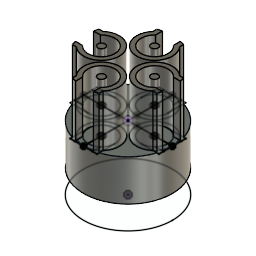
hexbug_circle_station (Autodesk Fusion 360 design; units mm, degrees)
Autodesk Fusion 360 part; units mm, degrees
note: some values were not read from the file. Set by a fixed rule: which sketch regions a step uses.
sketch "Sketch1" plane through (0, 0, 0) normal (0, 0, 1) x (1, 0, 0)
  circle A0 centre (0, 0) radius 12.45
  dimension "d1" = 24.9
  constraint coincident A0.centre origin
  measures "d1" diameter of A0
extrude "Extrude1" add sketch "Sketch1" along normal blind 18
sketch "Sketch2" plane through (0, 0, 18) normal (0, 0, 1) x (-1, 0, 0)
  circle A0 centre (0, 0) radius 12.45
  line L0 (0, 0) -> (0, -12.45)
  line L1 (0, 0) -> (-12.45, 0)
  line L2 (0, 0) -> (0, 12.45)
  line L3 (0, 0) -> (12.45, 0)
  line L4 (-12.45, 0) -> (-2.45, 0)
  circle A1 centre (-7.45, 0) radius 5
  line L5 (12.45, 0) -> (2.45, 0)
  line L6 (0, 12.45) -> (0, 2.45)
  line L7 (0, -12.45) -> (0, -2.45)
  circle A2 centre (0, -7.45) radius 5
  circle A3 centre (7.45, 0) radius 5
  circle A4 centre (0, 7.45) radius 5
  circle A5 centre (-7.45, 0) radius 3.75
  circle A6 centre (0, -7.45) radius 3.75
  circle A7 centre (0, 7.45) radius 3.75
  circle A8 centre (7.45, 0) radius 3.75
  circle A9 centre (-7.45, 0) radius 1
  circle A10 centre (0, -7.45) radius 1
  circle A11 centre (0, 7.45) radius 1
  circle A12 centre (7.45, 0) radius 1
  line L8 (-12.45, 0) -> (-12.45, -2.5)
  line L9 (-12.45, 0) -> (-12.45, 2.5)
  line L10 (-12.45, 2.5) -> (-11.7801, 2.5)
  line L11 (-12.45, -2.5) -> (-11.7801, -2.5)
  line L12 (0, -12.45) -> (-2.5, -12.45)
  line L13 (0, -12.45) -> (2.5, -12.45)
  line L14 (-2.5, -12.45) -> (-2.5, -11.7801)
  line L15 (12.45, 0) -> (12.45, -2.5)
  line L16 (12.45, 0) -> (12.45, 2.5)
  line L17 (12.45, 2.5) -> (10.2451, 2.5)
  line L18 (12.45, -2.5) -> (10.2451, -2.5)
  line L19 (2.5, -12.45) -> (2.5, -11.7801)
  line L20 (-2.5, -12.45) -> (-3.75, -12.45)
  line L21 (-3.75, -12.45) -> (-3.75, -10.7572)
  line L22 (2.5, -12.45) -> (3.75, -12.45)
  line L23 (3.75, -12.45) -> (3.75, -10.7572)
  line L24 (-3.75, -10.7572) -> (-3.75, -7.45)
  line L25 (2.5, -11.7801) -> (2.5, -10.2451)
  line L26 (-2.5, -11.7801) -> (-2.5, -10.2451)
  line L27 (3.75, -10.7572) -> (3.75, -7.45)
  line L28 (12.45, -2.5) -> (12.45, -3.75)
  line L29 (12.45, -3.75) -> (7.45, -3.75)
  line L30 (12.45, 1.25) -> (12.45, 2.5)
  line L31 (12.45, 2.5) -> (10.2451, 2.5)
  line L32 (12.45, 2.5) -> (12.45, 3.75)
  line L33 (12.45, 3.75) -> (7.45, 3.75)
  line L34 (0, 12.45) -> (-2.5, 12.45)
  line L35 (0, 12.45) -> (2.5, 12.45)
  line L36 (2.5, 12.45) -> (2.5, 10.2451)
  line L37 (2.5, 12.45) -> (3.75, 12.45)
  line L38 (3.75, 12.45) -> (3.75, 7.45)
  line L39 (-3.75, 7.45) -> (-3.75, 12.45)
  line L40 (-3.75, 12.45) -> (-2.5, 12.45)
  line L41 (-2.5, 12.45) -> (-2.5, 10.2451)
  line L42 (-11.7801, 2.5) -> (-10.2451, 2.5)
  line L43 (-11.7801, -2.5) -> (-10.2451, -2.5)
  line L44 (-12.45, -2.5) -> (-12.45, -3.75)
  line L45 (-12.45, 2.5) -> (-12.45, 3.75)
  line L46 (-12.45, 3.75) -> (-7.45, 3.75)
  line L47 (-12.45, -3.75) -> (-7.45, -3.75)
  dimension "d4" = 10
  dimension "d5" = 10
  dimension "d6" = 10
  dimension "d7" = 10
  dimension "d8" = 7.5
  dimension "d9" = 7.5
  dimension "d10" = 7.5
  dimension "d11" = 7.5
  dimension "d12" = 2
  dimension "d13" = 2
  dimension "d14" = 2
  dimension "d15" = 2
  dimension "d16" = 2.5
  dimension "d17" = 2.5
  dimension "d18" = 2.5
  dimension "d19" = 2.5
  dimension "d20" = 2.5
  dimension "d21" = 2.5
  dimension "d22" = 1.25
  dimension "d23" = 1.25
  dimension "d24" = 1.25
  dimension "d26" = 1.25
  dimension "d31" = 2.5
  dimension "d32" = 2.5
  dimension "d33" = 1.25
  dimension "d36" = 1.25
  dimension "d37" = 1.25
  constraint coincident A0.centre L0.start
  constraint coincident A0 L0.end
  constraint vertical L0
  constraint coincident A0 L1.end
  constraint perpendicular L0 L1
  constraint coincident A0 L2.end
  constraint perpendicular L1 L2
  constraint coincident A0 L3.end
  constraint perpendicular L2 L3
  constraint parallel L1 L4
  constraint midpoint L4 A1.centre
  constraint coincident L1.end A1
  constraint parallel L3 L5
  constraint parallel L2 L6
  constraint parallel L0 L7
  constraint midpoint L7 A2.centre
  constraint coincident L0.end A2
  constraint midpoint L5 A3.centre
  constraint coincident L3.end A3
  constraint midpoint L6 A4.centre
  constraint coincident L6.end A4
  constraint concentric A1 A5
  constraint concentric A2 A6
  constraint concentric A4 A7
  constraint concentric A3 A8
  constraint concentric A1 A9
  constraint concentric A6 A10
  constraint concentric A7 A11
  constraint concentric A8 A12
  constraint perpendicular L1 L8
  constraint perpendicular L1 L9
  constraint coincident A1 L10.end
  constraint perpendicular L9 L10
  constraint coincident A1 L11.end
  constraint perpendicular L8 L11
  constraint perpendicular L0 L12
  constraint perpendicular L0 L13
  constraint coincident A2 L14.end
  constraint perpendicular L12 L14
  constraint perpendicular L3 L15
  constraint perpendicular L3 L16
  constraint coincident A8 L17.end
  constraint perpendicular L16 L17
  constraint coincident A8 L18.end
  constraint perpendicular L15 L18
  constraint coincident A2 L19.end
  constraint perpendicular L13 L19
  constraint perpendicular L14 L20
  constraint coincident A2 L21.end
  constraint perpendicular L20 L21
  constraint perpendicular L19 L22
  constraint coincident A2 L23.end
  constraint perpendicular L22 L23
  constraint coincident A6 L24.end
  constraint tangent A6 L24
  constraint coincident A6 L25.end
  constraint parallel L19 L25
  constraint coincident A6 L26.end
  constraint parallel L14 L26
  constraint coincident A6 L27.end
  constraint tangent A6 L27
  constraint perpendicular L18 L28
  constraint coincident A8 L29.end
  constraint tangent A8 L29
  constraint midpoint L16 L30.start
  constraint perpendicular L29 L30
  constraint perpendicular L17 L32
  constraint coincident A8 L33.end
  constraint tangent A8 L33
  constraint perpendicular L32 L33
  constraint perpendicular L6 L34
  constraint tangent A0 L35
  constraint coincident A7 L36.end
  constraint perpendicular L35 L36
  constraint perpendicular L36 L37
  constraint coincident A7 L38.end
  constraint tangent A7 L38
  constraint coincident A7 L39.start
  constraint tangent A7 L39
  constraint parallel L38 L39
  constraint perpendicular L39 L40
  constraint coincident A7 L41.end
  constraint perpendicular L40 L41
  constraint coincident A5 L42.end
  constraint parallel L10 L42
  constraint coincident A5 L43.end
  constraint parallel L11 L43
  constraint perpendicular L11 L44
  constraint perpendicular L10 L45
  constraint coincident A5 L46.end
  constraint tangent A5 L46
  constraint coincident A5 L47.end
  constraint tangent A5 L47
  measures "d4" distance of L1.end L4.end
  measures "d5" distance of L3.end L5.end
  measures "d6" distance of L2.end L6.end
  measures "d7" distance of L0.end L7.end
  measures "d8" diameter of A5
  measures "d9" diameter of A6
  measures "d10" diameter of A7
  measures "d11" diameter of A8
  measures "d12" diameter of A9
  measures "d13" diameter of A10
  measures "d14" diameter of A11
  measures "d15" diameter of A12
  measures "d16" distance of L1.end L8.end
  measures "d17" distance of L1.end L9.end
  measures "d18" distance of L0.end L12.end
  measures "d19" distance of L0.end L13.end
  measures "d20" distance of L3.end L15.end
  measures "d21" distance of L3.end L16.end
  measures "d22" distance of L12.end L20.end
  measures "d23" distance of L13.end L22.end
  measures "d24" distance of L15.end L28.end
  measures "d26" distance of L16.end L32.end
  measures "d31" distance of L2.end L34.end
  measures "d32" distance of L2.end L35.end
  measures "d33" distance of L35.end L37.end
  measures "d36" distance of L8.end L44.end
  measures "d37" distance of L9.end L45.end
extrude "Extrude2" add sketch "Sketch2" along normal blind 14.44 contours A0 A2 L19 L23 | L0 L7 A2 A6 L27 | A2 A6 L25 L27 | L0 L7 A2 A6 L24 | A0 A2 L14 L21 | A2 A6 L24 L26 | L0 L7 A10 | L0 L7 A10
extrude "Extrude3" add sketch "Sketch2" along normal blind 14.44 contours A0 A3 L17 L31 L33 | A0 A3 L18 L29 | A3 A8 L17 L31 L33 | A3 A8 L18 L29 | L3 L5 A12 | L3 L5 A12 | L3 L5 A3 A8 L33 | L3 L5 A3 A8 L29
extrude "Extrude4" add sketch "Sketch2" along normal blind 14.44 contours A0 A4 L36 L38 | A4 A7 L36 L38 | L2 L6 A4 A7 L38 | L2 L6 A4 A7 L39 | A0 A4 L39 L41 | A4 A7 L39 L41 | L2 L6 A11 | L2 L6 A11
extrude "Extrude5" add sketch "Sketch2" along normal blind 14.44 contours L1 L4 A1 A5 L47 | L1 L4 A1 A5 L46 | A1 A5 L42 L46 | A0 A1 L10 L46 | A0 A1 L11 L47 | A1 A5 L43 L47 | L1 L4 A9 | L1 L4 A9
extrude "Extrude6" cut sketch "Sketch1" along normal blind 5
extrude "Extrude7" cut 1 faces at (3.0323, -6.4892, 5) along direction (0, 0, 1) blind 1.5
